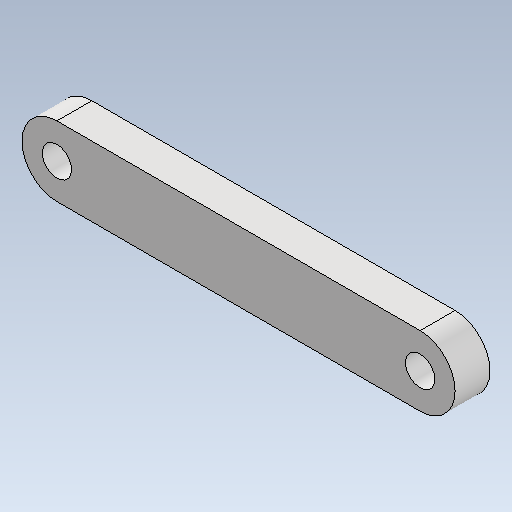
# Autodesk Inventor part: lower-tipper-link
Saved by Autodesk Inventor 2025 (Build 290162000, 162)
## iProperties
Created: 2025-08-20
Part Number: lower-tipper-link
Material: Generic
Document SubType Name: Modeling
Designer: HP
Density: 1 g/cm^3
Appearance: Default
Author: HP
Autodesk Inventor part; units mm, degrees
ref_plane "YZ Plane" through (0, 0, 0) normal (1, 0, 0) x (0, 1, 0)
ref_plane "XZ Plane" through (0, 0, 0) normal (0, 1, 0) x (-1, 0, 0)
ref_plane "XY Plane" through (0, 0, 0) normal (0, 0, 1) x (1, 0, 0)
sketch "Sketch1" plane through (0, 0, 0) normal (0, 0, 1) x (1, 0, 0)
  line L0 (-26, 0) -> (26, 0) construction
  line L1 (-26, -5) -> (26, -5)
  line L2 (26, 5) -> (-26, 5)
  arc A0 (-26, 5) -> (-26, -5) centre (-26, 0) ccw
  arc A1 (26, -5) -> (26, 5) centre (26, 0) ccw
  circle A2 centre (-26, 0) radius 2.1
  circle A3 centre (26, 0) radius 2.1
  point P0 (0, 0)
  point P1 (0, 0)
  point P2 (0, -1.8466)
  point P3 (0, 1.8466)
  dimension "d0" = 10
  dimension "d1" = 52
  dimension "d2" = 4.2
  dimension "d3" = 4.2
  constraints: 8 end point, 4 centre point, 4 point on circle, 4 tangent, 3 coincident, 1 horizontal, 1 midpoint, 1 parallel
  measures "d0" distance between parallel lines of L1 L2
  measures "d1" distance of L0.start L0.end
  measures "d2" diameter of A2
  measures "d3" diameter of A3
extrude "Extrusion1" add sketch "Sketch1" along normal blind 5
equation "\"d2\" = d3"
body "Solid1"
